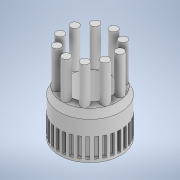
# Autodesk Inventor part: piece_roue_test_5
Saved by Autodesk Inventor 2020.1 (Build 241239000, 239)
## iProperties
Created: 2019-07-25
Part Number: piece_roue_test_5
Material: Générique
Document SubType Name: Modeling
Designer: marlo
Density: 1 g/cm^3
Appearance: Par défaut
Author: marlo
Autodesk Inventor part; units mm, degrees
ref_plane "YZ Plane" through (0, 0, 0) normal (1, 0, 0) x (0, 1, 0)
ref_plane "XZ Plane" through (0, 0, 0) normal (0, 1, 0) x (-1, 0, 0)
ref_plane "XY Plane" through (0, 0, 0) normal (0, 0, 1) x (1, 0, 0)
sketch "Esquisse2" plane through (0, 0, 0) normal (0, 1, 0) x (-1, 0, 0)
  circle A0 centre (0, 0) radius 18.5
  circle A1 centre (0, 0) radius 13.1
  dimension "d0" = 37
  dimension "d1" = 26.2
  constraints: 2 centre point, 2 coincident
  measures "d0" diameter of A0
  measures "d1" diameter of A1
extrude "Extrusion1" add sketch "Esquisse2" against normal blind 13
sketch "Esquisse3" plane through (0, 0, 0) normal (0, 1, 0) x (1, 0, 0)
  circle A0 centre (0, -15.8) radius 2.7
  line L0 (-22, 0) -> (25, 0) construction
  line L1 (-20, -18.5) -> (14, -18.5) construction
  circle A1 centre (0, 0) radius 18.5 construction
  circle A2 centre (-15.0267, 4.8825) radius 2.7
  line L2 (0, -15.8) -> (0, 0) construction
  line L3 (-15.0267, 4.8825) -> (0, 0) construction
  circle A3 centre (-15.0267, -4.8825) radius 2.7
  line L4 (0, 0) -> (-15.0267, -4.8825) construction
  line L5 (-15.0267, -4.8825) -> (-15.0267, 4.8825) construction
  line L6 (0, -31) -> (0, 24) construction
  line L7 (-15.0267, -4.8825) -> (-15.0267, -7.5825) construction
  line L8 (-15.0267, 4.8825) -> (-16.4693, 2.6002) construction
  line L9 (0, -15.8) -> (-2.3383, -17.15) construction
  circle A4 centre (-9.287, 12.7825) radius 2.7
  line L10 (0, 0) -> (-9.287, 12.7825) construction
  line L11 (-9.287, 12.7825) -> (-15.0267, 4.8825) construction
  line L12 (-9.287, 12.7825) -> (-7.7, 14.9668) construction
  circle A5 centre (-9.287, -12.7825) radius 2.7
  line L13 (-9.287, -12.7825) -> (0, 0) construction
  line L14 (-9.287, -12.7825) -> (0, -15.8) construction
  line L15 (-9.287, -12.7825) -> (-11.2119, -10.8891) construction
  line L16 (-9.287, -12.7825) -> (-15.0267, -4.8825) construction
  circle A6 centre (0, 15.8) radius 2.7
  line L17 (0, 15.8) -> (-1.5986, 17.9759) construction
  line L18 (0, 15.8) -> (0, 0) construction
  line L19 (0, 15.8) -> (-9.287, 12.7825) construction
  circle A7 centre (15.0267, 4.8825) radius 2.7
  circle A8 centre (15.0267, -4.8825) radius 2.7
  circle A9 centre (9.287, 12.7825) radius 2.7
  circle A10 centre (9.287, -12.7825) radius 2.7
  dimension "d4" = 5.4
  constraints: 40 end point, 14 equal length, 4 centre point, 4 symmetric about line, 3 horizontal, 3 point on line, 3 vertical, 1 coincident, 1 tangent, 1 vertical alignment, 21 other
extrude "Extrusion2" add sketch "Esquisse3" along normal blind 25
sketch "Esquisse4" plane through (0, -13, 0) normal (0, -1, 0) x (1, 0, 0)
  circle A0 centre (0, 0) radius 20.5
  circle A1 centre (0, 0) radius 13.1 projected
  circle A2 centre (0, 0) radius 18.5 projected
  circle A3 centre (0, 0) radius 13.1
  dimension "d9" = 2
  constraints: 2 centre point, 2 concentric, 1 coincident
  measures "d9" radial gap between concentric circles of A2 A0
extrude "Extrusion3" add sketch "Esquisse4" along normal blind 15 contours A0 | A2
sketch "Esquisse6" plane through (0, -13, 0) normal (0, 1, 0) x (1, 0, 0)
  arc A0 (-2, -20.4022) -> (0, -20.5) centre (0, 0) ccw
  circle A1 centre (0, 0) radius 20.5 construction
  line L0 (0, -20.5) -> (0, -18.5)
  line L1 (0, -36.4443) -> (0, 21.5557) construction
  circle A2 centre (0, 0) radius 18.5
  line L2 (-2, -20.4022) -> (-2, -18.3916)
  arc A3 (-10.874, -14.9668) -> (0, -18.5) centre (0, 0) ccw construction
  circle A4 centre (0, 0) radius 18.5 construction
  arc A5 (-2, -18.3916) -> (0, -18.5) centre (0, 0) ccw
  line L3 (0, 0) -> (-4.7726, -32.2215)
  arc A6 (-5.9425, -19.6198) -> (-4, -20.106) centre (0, 0) ccw
  line L4 (-5.9425, -19.6198) -> (-5.3627, -17.7057)
  line L5 (-4, -20.106) -> (-3.4172, -18.1817)
  arc A7 (-5.3627, -17.7057) -> (-3.4172, -18.1817) centre (0, 0) ccw
  line L6 (0, 0) -> (-10.8797, -30.4242)
  arc A8 (-12.9993, -15.8514) -> (-11.3908, -17.044) centre (0, 0) ccw
  line L7 (-12.9993, -15.8514) -> (-11.7311, -14.3049)
  line L8 (-11.3908, -17.044) -> (-10.1159, -15.4893)
  arc A9 (-11.7311, -14.3049) -> (-10.1159, -15.4893) centre (0, 0) ccw
  line L9 (-9.6565, -18.0832) -> (-8.887, -16.2257)
  line L10 (-7.8462, -18.939) -> (-7.0807, -17.0913)
  arc A10 (-9.6565, -18.0832) -> (-7.8462, -18.939) centre (0, 0) ccw
  arc A11 (-8.887, -16.2257) -> (-7.0807, -17.0913) centre (0, 0) ccw
  line L11 (0, 0) -> (-22.6613, -25.0088)
  arc A12 (-20.4008, -2.0141) -> (-20.107, -3.9948) centre (0, 0) ccw
  line L12 (-20.4008, -2.0141) -> (-18.4105, -1.8176)
  line L13 (-20.107, -3.9948) -> (-18.1061, -3.7973)
  arc A13 (-18.4105, -1.8176) -> (-18.1061, -3.7973) centre (0, 0) ccw
  line L14 (-19.6157, -5.956) -> (-17.758, -5.187)
  line L15 (-18.941, -7.8413) -> (-17.0931, -7.0763)
  arc A14 (-19.6157, -5.956) -> (-18.941, -7.8413) centre (0, 0) ccw
  arc A15 (-17.758, -5.187) -> (-17.0931, -7.0763) centre (0, 0) ccw
  line L16 (-18.0765, -9.669) -> (-16.313, -8.7257)
  line L17 (-17.047, -11.3864) -> (-15.274, -10.4381)
  arc A16 (-18.0765, -9.669) -> (-17.047, -11.3864) centre (0, 0) ccw
  arc A17 (-16.313, -8.7257) -> (-15.274, -10.4381) centre (0, 0) ccw
  arc A18 (-15.8424, -13.0103) -> (-14.4976, -14.4938) centre (0, 0) ccw
  line L18 (-14.4976, -14.4938) -> (-13.0832, -13.0798)
  line L19 (-15.8424, -13.0103) -> (-14.4205, -11.5887)
  arc A19 (-14.4205, -11.5887) -> (-13.0832, -13.0798) centre (0, 0) ccw
  circle A20 centre (0, 0) radius 20.5 projected
  line L20 (-7.8462, -18.939) -> (-5.9425, -19.6198) construction
  line L21 (-2, -20.4022) -> (-4, -20.106) construction
  line L22 (-14.4976, -14.4938) -> (-12.9993, -15.8514) construction
  line L23 (0, 0) -> (-28.6008, -1.4047)
  arc A21 (-2.0088, 20.4013) -> (-3.9896, 20.108) centre (0, 0) ccw
  line L24 (-2.0088, 20.4013) -> (-1.8128, 18.411)
  line L25 (-3.9896, 20.108) -> (-3.7926, 18.1071)
  arc A22 (-1.8128, 18.411) -> (-12.2883, 13.8292) centre (0, 0) ccw construction
  arc A23 (-1.8128, 18.411) -> (-3.7926, 18.1071) centre (0, 0) ccw
  line L26 (-5.951, 19.6172) -> (-5.1824, 17.7593)
  line L27 (-7.8365, 18.9431) -> (-7.0719, 17.095)
  arc A24 (-5.951, 19.6172) -> (-7.8365, 18.9431) centre (0, 0) ccw
  arc A25 (-5.1824, 17.7593) -> (-7.0719, 17.095) centre (0, 0) ccw
  line L28 (-9.6643, 18.079) -> (-8.7215, 16.3152)
  line L29 (-11.382, 17.0499) -> (-10.4342, 15.2767)
  arc A26 (-9.6643, 18.079) -> (-11.382, 17.0499) centre (0, 0) ccw
  arc A27 (-8.7215, 16.3152) -> (-10.4342, 15.2767) centre (0, 0) ccw
  arc A28 (-13.0062, 15.8458) -> (-14.4901, 14.5013) centre (0, 0) ccw
  line L30 (-14.4901, 14.5013) -> (-13.0764, 13.0865)
  line L31 (-13.0062, 15.8458) -> (-11.585, 14.4235)
  arc A29 (-11.585, 14.4235) -> (-13.0764, 13.0865) centre (0, 0) ccw
  arc A30 (-17.7043, 5.3673) -> (-18.1808, 3.4219) centre (0, 0) ccw
  arc A31 (-16.2234, 8.8911) -> (-17.0895, 7.0852) centre (0, 0) ccw
  arc A32 (-14.3019, 11.7348) -> (-15.4867, 10.1199) centre (0, 0) ccw
  line L32 (-20.5, 0.0053) -> (-18.5, 0.0048)
  line L33 (-20.4017, 2.0053) -> (-18.3911, 2.0047)
  line L34 (-20.1049, 4.0052) -> (-18.1808, 3.4219)
  arc A33 (-19.6183, 5.9475) -> (-20.1049, 4.0052) centre (0, 0) ccw
  line L35 (-19.6183, 5.9475) -> (-17.7043, 5.3673)
  line L36 (-18.937, 7.8511) -> (-17.0895, 7.0852)
  line L37 (-17.0411, 11.3952) -> (-15.4867, 10.1199)
  line L38 (-18.0807, 9.6612) -> (-16.2234, 8.8911)
  arc A34 (-15.8481, 13.0034) -> (-17.0411, 11.3952) centre (0, 0) ccw
  arc A35 (-18.0807, 9.6612) -> (-18.937, 7.8511) centre (0, 0) ccw
  arc A36 (-20.4017, 2.0053) -> (-20.5, 0.0053) centre (0, 0) ccw
  arc A37 (-18.3911, 2.0047) -> (-18.5, 0.0048) centre (0, 0) ccw
  line L39 (-15.8481, 13.0034) -> (-14.3019, 11.7348)
  line L40 (-9.6643, 18.079) -> (-7.8365, 18.9431) construction
  line L41 (-3.9896, 20.108) -> (-5.951, 19.6172) construction
  line L42 (-15.8481, 13.0034) -> (-14.4901, 14.5013) construction
  line L43 (-20.5, 0.0053) -> (-20.4008, -2.0141)
  line L44 (0, 0) -> (-1.4431, 29.5374)
  arc A38 (1.9983, -20.4024) -> (3.9792, -20.1101) centre (0, 0) ccw
  line L45 (1.9983, -20.4024) -> (1.8033, -18.4119)
  line L46 (3.9792, -20.1101) -> (3.7833, -18.109)
  arc A39 (1.8033, -18.4119) -> (12.2812, -13.8356) centre (0, 0) ccw construction
  arc A40 (1.8033, -18.4119) -> (3.7833, -18.109) centre (0, 0) ccw
  line L47 (5.9408, -19.6203) -> (5.1732, -17.762)
  line L48 (7.8267, -18.9471) -> (7.0631, -17.0986)
  arc A41 (5.9408, -19.6203) -> (7.8267, -18.9471) centre (0, 0) ccw
  arc A42 (5.1732, -17.762) -> (7.0631, -17.0986) centre (0, 0) ccw
  line L49 (9.655, -18.084) -> (8.7131, -16.3197)
  line L50 (11.3732, -17.0558) -> (10.4263, -15.2821)
  arc A43 (9.655, -18.084) -> (11.3732, -17.0558) centre (0, 0) ccw
  arc A44 (8.7131, -16.3197) -> (10.4263, -15.2821) centre (0, 0) ccw
  arc A45 (12.998, -15.8525) -> (14.4826, -14.5088) centre (0, 0) ccw
  line L51 (14.4826, -14.5088) -> (13.0697, -13.0933)
  line L52 (12.998, -15.8525) -> (11.5776, -14.4295)
  arc A46 (11.5776, -14.4295) -> (13.0697, -13.0933) centre (0, 0) ccw
  arc A47 (17.7015, -5.3764) -> (18.179, -3.4312) centre (0, 0) ccw
  arc A48 (16.2188, -8.8995) -> (17.0858, -7.094) centre (0, 0) ccw
  arc A49 (14.2959, -11.7422) -> (15.4815, -10.1279) centre (0, 0) ccw
  line L53 (20.5, -0.0159) -> (18.5, -0.0143)
  line L54 (20.4007, -2.0158) -> (18.39, -2.0142)
  line L55 (20.1029, -4.0156) -> (18.179, -3.4312)
  arc A50 (19.6152, -5.9577) -> (20.1029, -4.0156) centre (0, 0) ccw
  line L56 (19.6152, -5.9577) -> (17.7015, -5.3764)
  line L57 (18.9329, -7.8609) -> (17.0858, -7.094)
  line L58 (17.0352, -11.404) -> (15.4815, -10.1279)
  line L59 (18.0757, -9.6705) -> (16.2188, -8.8995)
  arc A51 (15.8414, -13.0116) -> (17.0352, -11.404) centre (0, 0) ccw
  arc A52 (18.0757, -9.6705) -> (18.9329, -7.8609) centre (0, 0) ccw
  arc A53 (20.4007, -2.0158) -> (20.5, -0.0159) centre (0, 0) ccw
  arc A54 (18.39, -2.0142) -> (18.5, -0.0143) centre (0, 0) ccw
  line L60 (15.8414, -13.0116) -> (14.2959, -11.7422)
  line L61 (9.655, -18.084) -> (7.8267, -18.9471) construction
  line L62 (3.9792, -20.1101) -> (5.9408, -19.6203) construction
  line L63 (15.8414, -13.0116) -> (14.4826, -14.5088) construction
  arc A55 (2.0105, 20.4012) -> (0.0106, 20.5) centre (0, 0) ccw
  arc A56 (2.0095, 18.3905) -> (0.0095, 18.5) centre (0, 0) ccw
  arc A57 (10.8817, 14.9612) -> (0.0095, 18.5) centre (0, 0) ccw construction
  line L64 (17.0528, 11.3776) -> (15.2794, 10.4302)
  arc A58 (16.3175, 8.7173) -> (15.2794, 10.4302) centre (0, 0) ccw
  line L65 (18.0815, 9.6597) -> (16.3175, 8.7173)
  arc A59 (17.7606, 5.1778) -> (17.0968, 7.0675) centre (0, 0) ccw
  arc A60 (19.6188, 5.9459) -> (18.9451, 7.8316) centre (0, 0) ccw
  line L66 (19.6188, 5.9459) -> (17.7606, 5.1778)
  arc A61 (18.4114, 1.8081) -> (18.1081, 3.7879) centre (0, 0) ccw
  line L67 (20.4019, 2.0036) -> (18.4114, 1.8081)
  line L68 (2.0105, 20.4012) -> (2.0095, 18.3905)
  line L69 (0.0106, 20.5) -> (0.0095, 18.5)
  line L70 (20.1091, 3.9844) -> (18.1081, 3.7879)
  arc A62 (18.0815, 9.6597) -> (17.0528, 11.3776) centre (0, 0) ccw
  line L71 (18.9451, 7.8316) -> (17.0968, 7.0675)
  line L72 (11.3996, 17.0381) -> (10.1239, 15.4841)
  arc A63 (11.7385, 14.2989) -> (10.1239, 15.4841) centre (0, 0) ccw
  arc A64 (13.0075, 15.8447) -> (11.3996, 17.0381) centre (0, 0) ccw
  line L73 (13.0075, 15.8447) -> (11.7385, 14.2989)
  line L74 (14.505, 14.4863) -> (13.0075, 15.8447) construction
  line L75 (14.505, 14.4863) -> (13.0899, 13.073)
  arc A65 (14.4265, 11.5813) -> (13.0899, 13.073) centre (0, 0) ccw
  arc A66 (15.8491, 13.0021) -> (14.505, 14.4863) centre (0, 0) ccw
  line L76 (15.8491, 13.0021) -> (14.4265, 11.5813)
  line L77 (4.0104, 20.1039) -> (3.4265, 18.1799)
  arc A67 (8.8953, 16.2211) -> (7.0896, 17.0877) centre (0, 0) ccw
  arc A68 (9.6658, 18.0782) -> (7.856, 18.935) centre (0, 0) ccw
  line L78 (7.856, 18.935) -> (7.0896, 17.0877)
  line L79 (7.856, 18.935) -> (5.9526, 19.6167) construction
  line L80 (5.9526, 19.6167) -> (5.3719, 17.7029)
  arc A69 (5.3719, 17.7029) -> (3.4265, 18.1799) centre (0, 0) ccw
  arc A70 (5.9526, 19.6167) -> (4.0104, 20.1039) centre (0, 0) ccw
  line L81 (2.0105, 20.4012) -> (4.0104, 20.1039) construction
  line L82 (9.6658, 18.0782) -> (8.8953, 16.2211)
  arc A71 (20.4019, 2.0036) -> (20.1091, 3.9844) centre (0, 0) ccw
  line L83 (20.4019, 2.0036) -> (20.5, -0.0159)
  line L84 (-2.0088, 20.4013) -> (0.0106, 20.5) construction
  point P0 (-2, -18.3916)
  point P1 (-2.1012, 21.4531)
  point P2 (-13.0832, -13.0798)
  point P3 (-14.4205, -11.5887)
  point P4 (-15.274, -10.4381)
  point P5 (-16.313, -8.7257)
  point P6 (-17.0931, -7.0763)
  point P7 (-17.758, -5.187)
  point P8 (-18.3911, 2.0047)
  point P9 (-18.5, 0.0048)
  point P10 (-17.7043, 5.3673)
  point P11 (-19.6183, 5.9475)
  point P12 (-20.1049, 4.0052)
  point P13 (-18.1808, 3.4219)
  point P14 (-17.0895, 7.0852)
  point P15 (-17.0411, 11.3952)
  point P16 (-15.4867, 10.1199)
  point P17 (-14.4901, 14.5013)
  point P18 (-13.0764, 13.0865)
  point P19 (-11.382, 17.0499)
  point P20 (-10.4342, 15.2767)
  point P21 (-8.7215, 16.3152)
  point P22 (-9.6643, 18.079)
  point P23 (0.0106, 20.5)
  point P24 (0.0095, 18.5)
  point P25 (2.0095, 18.3905)
  point P26 (2.0105, 20.4012)
  point P27 (4.0104, 20.1039)
  point P28 (3.4265, 18.1799)
  point P29 (16.3175, 8.7173)
  point P30 (14.4265, 11.5813)
  point P31 (15.8491, 13.0021)
  point P32 (11.3996, 17.0381)
  point P33 (10.1239, 15.4841)
  point P34 (11.7385, 14.2989)
  point P35 (7.0896, 17.0877)
  point P36 (-1.8128, 18.411)
  point P37 (-2.0088, 20.4013)
  point P38 (-3.9896, 20.108)
  point P39 (-3.7926, 18.1071)
  point P40 (3.9792, -20.1101)
  point P41 (5.1732, -17.762)
  point P42 (5.9408, -19.6203)
  point P43 (7.0631, -17.0986)
  point P44 (11.3732, -17.0558)
  point P45 (10.4263, -15.2821)
  point P46 (9.655, -18.084)
  point P47 (13.0697, -13.0933)
  point P48 (17.0352, -11.404)
  point P49 (18.9329, -7.8609)
  point P50 (20.1029, -4.0156)
  point P51 (18.179, -3.4312)
  point P52 (18.1081, 3.7879)
  point P53 (17.0968, 7.0675)
  dimension "d17" = 2
  dimension "d24" = 2
  dimension "d25" = 2
  constraints: 167 end point, 128 symmetric about line, 10 point on circle, 4 centre point, 4 equal length, 2 coincident, 2 point on line, 2 vertical, 1 collinear, 1 concentric, 267 other
  measures "d17" horizontal distance of L0.start L2.start
  measures "d24" distance of L0.start L0.end
  measures "d25" horizontal distance of L2.start L5.start
extrude "Extrusion5" cut sketch "Esquisse6" against normal blind 15 contours L2 A2 L0 A0 | L45 A2 L46 A20 | A6 L4 A2 L5 | L47 A2 L48 A20 | L10 A10 L9 A2 | L18 A18 L19 A2 | A2 L8 A8 L7 | L32 A20 L33 A2 | A2 L13 A12 L12 | L69 A20 L68 A2 | A2 L25 A20 L24 | L49 A2 L50 A20 | L17 A16 L16 A2 | L34 A20 L35 A2 | A2 L15 A14 L14 | L77 A20 L80 A2 | A2 L27 A20 L26 | L52 A2 L51 A20 | L36 A20 L38 A2 | L78 A20 L82 A2 | A2 L29 A20 L28 | L60 A2 L58 A20 | L37 A20 L39 A2 | L72 A20 L73 A2 | A2 L30 A20 L31 | L59 A2 L57 A20 | L75 A20 L76 A2 | L56 A2 L55 A20 | L64 A20 L65 A2 | L54 A2 L53 A20 | L71 A20 L66 A2 | L67 A2 L70 A20
sketch "Esquisse7" plane through (0, -28, 0) normal (0, -1, 0) x (1, 0, 0)
  arc A0 (15.8414, 13.0116) -> (14.4826, 14.5088) centre (0, 0) ccw projected
  circle A1 centre (0, 0) radius 20.5
  circle A2 centre (0, 0) radius 13.1
  point P0 (15.8414, 13.0116)
  constraints: 2 coincident, 1 centre point, 3 other
extrude "Extrusion6" add sketch "Esquisse7" along normal blind 2
sketch "Esquisse8" plane through (0, 0, 0) normal (0, 1, 0) x (1, 0, 0)
  arc A0 (-8.887, -16.2257) -> (-7.0807, -17.0913) centre (0, 0) ccw projected
  circle A1 centre (0, 0) radius 18.5
  arc A2 (-9.6565, -18.0832) -> (-7.8462, -18.939) centre (0, 0) ccw projected
  circle A3 centre (0, 0) radius 20.5
  point P0 (-8.887, -16.2257)
  point P1 (-7.8462, -18.939)
  point P2 (-9.6565, -18.0832)
  constraints: 2 coincident, 1 centre point, 3 other
extrude "Extrusion7" add sketch "Esquisse8" against normal blind 15
chamfer "Chanfrein2" distance 2 distance2 5 2 edges at (8.7618, 0, -18.5332) (-8.7618, 0, 18.5332) measured on face at (8.5481, 0, -18.0812) measured on face at (-8.5481, 0, 18.0812)
